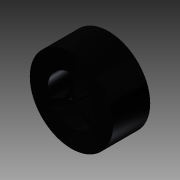
# Autodesk Inventor part: koleso
Saved by Autodesk Inventor 2015 (Build 190159000, 159)
## iProperties
Created: 2015-06-07
Part Number: koleso
Material: ABS Plastic
Document SubType Name: Modeling
Designer: Jufo
Density: 1 g/cm^3
Appearance: Smooth - White
Author: Jufo
Autodesk Inventor part; units mm, degrees
ref_plane "YZ Plane" through (0, 0, 0) normal (1, 0, 0) x (0, 1, 0)
ref_plane "XZ Plane" through (0, 0, 0) normal (0, 1, 0) x (-1, 0, 0)
ref_plane "XY Plane" through (0, 0, 0) normal (0, 0, 1) x (1, 0, 0)
sketch "Sketch1" plane through (0, 0, 0) normal (0, 1, 0) x (-1, 0, 0)
  circle A0 centre (0, 0) radius 45
  circle A1 centre (0, 0) radius 25.5
  dimension "d0" = 90
  dimension "d1" = 51
  constraints: 2 centre point, 2 coincident
  measures "d0" diameter of A0
  measures "d1" diameter of A1
extrude "Extrusion1" add sketch "Sketch1" along normal blind 40
sketch "Sketch2" plane through (0, 0, 0) normal (0, -1, 0) x (1, 0, 0)
  circle A0 centre (0, 0) radius 25.5 projected
  circle A1 centre (0, 0) radius 45 projected
  line L0 (6.2, 0) -> (3.1, -5.3694)
  line L1 (3.1, -5.3694) -> (-3.1, -5.3694)
  line L2 (-3.1, -5.3694) -> (-6.2, 0)
  line L3 (-6.2, 0) -> (-3.1, 5.3694)
  line L4 (-3.1, 5.3694) -> (3.1, 5.3694)
  line L5 (3.1, 5.3694) -> (6.2, 0)
  line L6 (-3.1, 5.3694) -> (-3.1, 25.3109)
  line L7 (3.1, 5.3694) -> (3.1, 25.3109)
  line L8 (6.2, 0) -> (23.4699, -9.9708)
  line L9 (3.1, -5.3694) -> (20.3699, -15.3401)
  line L10 (-3.1, -5.3694) -> (-20.3699, -15.3401)
  line L11 (-6.2, 0) -> (-23.4699, -9.9708)
  circle A2 centre (0, 0) radius 6.5
  dimension "d4" = 6.2
  dimension "d5" = 13
  constraints: 24 end point, 6 point on circle, 3 perpendicular, 2 coincident, 1 centre point, 13 other
  measures "d4" distance of L3.end L4.end
  measures "d5" diameter of A2
extrude "Extrusion2" add sketch "Sketch2" against normal blind 15 contours L7 A2 L6 A0 | A0 L9 A2 L8 | A2 L8 L5 L7 | L7 L4 L6 A2 | A2 L9 L0 L8 | L11 A2 L10 A0 | L6 L3 L11 A2 | A2 L10 L1 L9 | L11 L2 L10 A2
sketch "Sketch3" plane through (0, 0, 0) normal (0, -1, 0) x (1, 0, 0)
  line L0 (3.1, -5.3694) -> (-3.1, -5.3694) projected
  line L1 (-3.1, -5.3694) -> (-6.2, 0) projected
  line L2 (-6.2, 0) -> (-3.1, 5.3694) projected
  line L3 (-3.1, 5.3694) -> (3.1, 5.3694) projected
  line L4 (3.1, 5.3694) -> (6.2, 0) projected
  line L5 (6.2, 0) -> (3.1, -5.3694) projected
  circle A0 centre (0, 0) radius 45 projected
  circle A1 centre (0, 0) radius 2
  dimension "d8" = 4
  constraints: 1 centre point, 1 coincident
  measures "d8" diameter of A1
extrude "Extrusion3" add sketch "Sketch3" against normal blind 5 contours L0 L1 L2 L3 L4 L5
body "Solid1"
